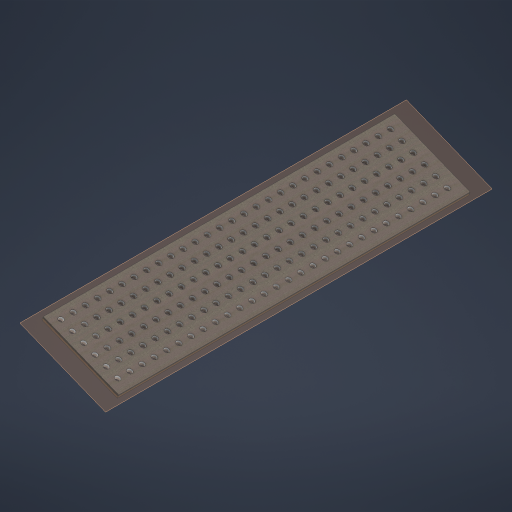
# Autodesk Inventor part: platte
Saved by Autodesk Inventor 2023 (Build 270158000, 158)
## iProperties
Created: 2022-06-24
Part Number: platte
Material: Generic
Document SubType Name: Modeling
Designer: bananenbrot
Density: 1 g/cm^3
Appearance: Default
Author: bananenbrot
Autodesk Inventor part; units mm, degrees
ref_plane "YZ Plane" through (0, 0, 0) normal (1, 0, 0) x (0, 1, 0)
ref_plane "XZ Plane" through (0, 0, 0) normal (0, 1, 0) x (-1, 0, 0)
ref_plane "XY Plane" through (0, 0, 0) normal (0, 0, 1) x (1, 0, 0)
ref_plane "Work Plane1" through (0, 0, 0) normal (0, 0, 1) x (1, 0, 0)
sketch "Sketch1" plane through (0, 0, 0) normal (0, 0, 1) x (1, 0, 0)
  arc A0 (11.7519, -6.4859) -> (17.0448, -5.0515) centre (7.6561, 19.1093) ccw projected
  line L0 (30.2513, -13.8976) -> (11.7519, -6.4859) projected
  line L1 (31.4786, -10.8344) -> (30.2513, -13.8976) projected
  line L2 (17.0448, -5.0515) -> (31.4786, -10.8344) projected
  arc A1 (-15.8175, 8.1147) -> (-12.9792, 3.4226) centre (7.6561, 19.1093) ccw projected
  line L3 (-30.2513, 13.8976) -> (-15.8175, 8.1147) projected
  line L4 (-31.4786, 10.8344) -> (-30.2513, 13.8976) projected
  line L5 (-12.9792, 3.4226) -> (-31.4786, 10.8344) projected
  line L6 (17.0448, -5.0515) -> (-15.8175, 8.1147)
  line L7 (11.7519, -6.4859) -> (-12.9792, 3.4226)
  point P0 (0, 0)
  constraints: 4 end point, 1 collinear
extrude "Extrusion1" add sketch "Sketch1" along normal blind 288
sketch "Sketch2" plane through (-30.2513, 13.8976, 288) normal (0.3719097, 0.9282689, 0) x (0.9282689, -0.3719097, 0)
  circle A0 centre (7.1485, 7.8489) radius 2
  point P0 (33.25, 288)
  dimension "d2" = 4
  constraints: 1 centre point
  measures "d2" diameter of A0
extrude "Extrusion2" cut sketch "Sketch2" against normal blind 288
pattern_linear "Rectangular Pattern1" count 28 spacing 10 along (0, 0, -1) count 6 spacing 10 along (0.9282689, -0.3719097, 0) of "Extrusion2"
ref_plane "Work Plane2" through (-30.8649, 12.366, 288) normal (0.3719097, 0.9282689, 0) x (0.9282689, -0.3719097, 0)
body "Solid1"
